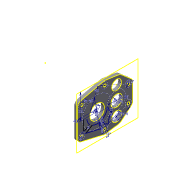
# Autodesk Inventor part: BackPlate
Saved by Autodesk Inventor 2013 SP1 (Build 170176100, 176)
## iProperties
Created: 2013-11-05
Part Number: BackPlate
Material: Generic
Document SubType Name: Modeling
Designer: robotics
Density: 1 g/cm^3
Author: robotics
Autodesk Inventor part; units mm, degrees
ref_plane "YZ Plane" through (0, 0, 0) normal (1, 0, 0) x (0, 1, 0)
ref_plane "XZ Plane" through (0, 0, 0) normal (0, 1, 0) x (-1, 0, 0)
ref_plane "XY Plane" through (0, 0, 0) normal (0, 0, 1) x (1, 0, 0)
sketch "Sketch1" plane through (0, 0, 0) normal (1, 0, 0) x (0, 1, 0)
  line L0 (181.2823, -83.3004) -> (61.2823, -83.3004)
  line L1 (61.2823, -83.3004) -> (61.2823, -183.3004)
  line L2 (61.2823, -183.3004) -> (181.2823, -183.3004)
  line L3 (181.2823, -183.3004) -> (181.2823, -83.3004)
  point P0 (0, 0)
  dimension "d0" = 100
  dimension "d2" = 120
  constraints: 8 end point, 2 parallel, 1 horizontal, 1 perpendicular, 1 other
  measures "d0" distance of L2.end L0.start
  measures "d2" distance of L0.start L0.end
extrude "Extrusion1" add sketch "Sketch1" along normal blind 6
sketch "Sketch2" plane through (6, 0, 0) normal (1, 0, 0) x (0, 0, -1)
  line L0 (83.3004, 181.2823) -> (83.3004, 61.2823) projected
  line L1 (83.3004, 61.2823) -> (183.3004, 61.2823) projected
  line L2 (183.3004, 61.2823) -> (183.3004, 181.2823) projected
  line L3 (183.3004, 181.2823) -> (83.3004, 181.2823) projected
  circle A0 centre (133.3004, 139.3823) radius 17.78 construction
  circle A1 centre (133.3004, 139.3823) radius 9.525 construction
  circle A2 centre (159.9704, 139.3823) radius 8.89 construction
  circle A3 centre (106.6304, 139.3823) radius 8.89 construction
  circle A4 centre (133.3004, 101.2823) radius 28.575 construction
  line L4 (159.9704, 139.3823) -> (149.536, 162.5401) construction
  line L5 (159.9704, 139.3823) -> (170.4047, 116.2245) construction
  line L6 (96.196, 116.2245) -> (106.6304, 139.3823) construction
  line L7 (106.6304, 139.3823) -> (117.0647, 162.5401) construction
  circle A5 centre (149.536, 162.5401) radius 6.35 construction
  circle A6 centre (170.4047, 116.2245) radius 6.35 construction
  circle A7 centre (96.196, 116.2245) radius 6.35 construction
  circle A8 centre (117.0647, 162.5401) radius 6.35 construction
  circle A9 centre (159.9704, 71.471) radius 6.35 construction
  circle A10 centre (106.6304, 71.471) radius 6.35 construction
  point P0 (0, 0)
  dimension "d5" = 35.56
  dimension "d7" = 19.05
  dimension "d8" = 57.15
  dimension "d9" = 17.78
  dimension "d10" = 25.4
  dimension "d11" = 12.7
  dimension "d12" = 40
  dimension "d13" = 40
  dimension "d14" = 50
  dimension "d22" = 40
  constraints: 11 centre point, 8 end point, 6 equal radius, 5 coincident, 4 horizontal alignment, 3 equal length, 3 tangent, 3 vertical alignment, 2 collinear
  measures "d5" diameter of A0
  measures "d7" diameter of A1
  measures "d8" diameter of A4
  measures "d9" diameter of A2
  measures "d10" distance of L4.start L4.end
  measures "d11" diameter of A8
  measures "d12" distance of A4.centre A7.centre
  measures "d13" distance from line of A4.centre L1
  measures "d14" distance from line of L0 A4.centre
  measures "d22" distance of A4.centre A10.centre
sketch "Sketch3" plane through (6, 0, 0) normal (1, 0, 0) x (0, 0, -1)
  circle A0 centre (133.3004, 101.2823) radius 14.2875
  circle A1 centre (133.3004, 139.3823) radius 11.1125
  circle A2 centre (106.6304, 139.3823) radius 9.5631
  circle A3 centre (159.9704, 139.3823) radius 9.5631
  circle A4 centre (170.4047, 116.2245) radius 2.5
  circle A5 centre (149.536, 162.5401) radius 2.5
  circle A6 centre (117.0647, 162.5401) radius 2.5
  circle A7 centre (96.196, 116.2245) radius 2.5
  circle A8 centre (106.6304, 71.471) radius 2.5
  circle A9 centre (159.9704, 71.471) radius 2.5
  point P0 (0, 0)
  dimension "d15" = 22.225
  dimension "d17" = 28.575
  dimension "d18" = 19.1262
  dimension "d19" = 5
  constraints: 10 centre point, 10 coincident, 6 equal radius
  measures "d15" diameter of A1
  measures "d17" diameter of A0
  measures "d18" diameter of A2
  measures "d19" diameter of A4
extrude "Extrusion2" cut sketch "Sketch3" against normal blind 6
sketch "Sketch4" plane through (6, 0, 0) normal (1, 0, 0) x (0, 0, -1)
  circle A0 centre (133.3004, 139.3823) radius 11.1125 projected
  circle A1 centre (170.4047, 116.2245) radius 2.5 projected
  circle A2 centre (149.536, 162.5401) radius 2.5 projected
  circle A3 centre (159.9704, 139.3823) radius 9.5631 projected
  circle A4 centre (133.3004, 101.2823) radius 14.2875 projected
  line L0 (83.3004, 181.2823) -> (83.3004, 61.2823) projected
  line L1 (83.3004, 61.2823) -> (183.3004, 61.2823) projected
  line L2 (183.3004, 61.2823) -> (183.3004, 181.2823) projected
  line L3 (183.3004, 181.2823) -> (83.3004, 181.2823) projected
  circle A5 centre (106.6304, 71.471) radius 2.5 projected
  circle A6 centre (159.9704, 71.471) radius 2.5 projected
  arc A7 (159.9704, 62.971) -> (168.2483, 69.541) centre (159.9704, 71.471) ccw
  arc A8 (178.6827, 114.2944) -> (178.8197, 117.4236) centre (170.4047, 116.2245) ccw
  arc A9 (175.3778, 141.5778) -> (171.8222, 149.4691) centre (159.9704, 139.3823) ccw
  arc A10 (156.0091, 168.0492) -> (149.536, 171.0401) centre (149.536, 162.5401) ccw
  line L4 (168.2483, 69.541) -> (178.6827, 114.2944)
  line L5 (178.8197, 117.4236) -> (175.3778, 141.5778)
  line L6 (171.8222, 149.4691) -> (156.0091, 168.0492)
  line L7 (149.536, 171.0401) -> (133.3004, 171.0401)
  line L8 (159.9704, 62.971) -> (133.3004, 62.971)
  line L9 (133.3004, 139.3823) -> (133.3004, 101.2823) construction
  arc A11 (98.3524, 69.541) -> (106.6304, 62.971) centre (106.6304, 71.471) ccw
  arc A12 (87.781, 117.4236) -> (87.918, 114.2944) centre (96.196, 116.2245) ccw
  arc A13 (94.7785, 149.4691) -> (91.2229, 141.5778) centre (106.6304, 139.3823) ccw
  arc A14 (117.0647, 171.0401) -> (110.5917, 168.0492) centre (117.0647, 162.5401) ccw
  line L10 (98.3524, 69.541) -> (87.918, 114.2944)
  line L11 (87.781, 117.4236) -> (91.2229, 141.5778)
  line L12 (94.7785, 149.4691) -> (110.5917, 168.0492)
  line L13 (117.0647, 171.0401) -> (133.3004, 171.0401)
  line L14 (106.6304, 62.971) -> (133.3004, 62.971)
  point P0 (0, 0)
  dimension "d23" = 6
  dimension "d24" = 6
  constraints: 22 end point, 16 point on circle, 12 symmetric about line, 8 centre point, 8 tangent, 4 coincident, 2 equal radius, 2 parallel, 2 vertical alignment, 1 perpendicular, 4 other
  measures "d23" radial gap between concentric circles of A7 A6
  measures "d24" radial gap between concentric circles of A3 A9
extrude "Extrusion3" cut sketch "Sketch4" against normal blind 6 contours L3 L2 L1 L0
sketch "Sketch7" plane through (6, 0, 0) normal (1, 0, 0) x (0, 0, -1)
  line L0 (168.2483, 69.541) -> (178.6827, 114.2944) projected
  arc A0 (178.6827, 114.2944) -> (178.8197, 117.4236) centre (170.4047, 116.2245) ccw projected
  line L1 (178.8197, 117.4236) -> (175.3778, 141.5778) projected
  arc A1 (175.3778, 141.5778) -> (171.8222, 149.4691) centre (159.9704, 139.3823) ccw projected
  line L2 (171.8222, 149.4691) -> (156.0091, 168.0492) projected
  arc A2 (156.0091, 168.0492) -> (149.536, 171.0401) centre (149.536, 162.5401) ccw projected
  line L3 (149.536, 171.0401) -> (117.0647, 171.0401) projected
  arc A3 (117.0647, 171.0401) -> (110.5917, 168.0492) centre (117.0647, 162.5401) ccw projected
  line L4 (110.5917, 168.0492) -> (94.7785, 149.4691) projected
  arc A4 (94.7785, 149.4691) -> (91.2229, 141.5778) centre (106.6304, 139.3823) ccw projected
  line L5 (91.2229, 141.5778) -> (87.781, 117.4236) projected
  arc A5 (87.781, 117.4236) -> (87.918, 114.2944) centre (96.196, 116.2245) ccw projected
  line L6 (87.918, 114.2944) -> (98.3524, 69.541) projected
  arc A6 (98.3524, 69.541) -> (106.6304, 62.971) centre (106.6304, 71.471) ccw projected
  line L7 (106.6304, 62.971) -> (159.9704, 62.971) projected
  arc A7 (159.9704, 62.971) -> (168.2483, 69.541) centre (159.9704, 71.471) ccw projected
  circle A8 centre (133.3004, 139.3823) radius 11.1125 projected
  circle A9 centre (106.6304, 139.3823) radius 9.5631 projected
  circle A10 centre (106.6304, 71.471) radius 2.5 projected
  circle A11 centre (117.0647, 162.5401) radius 2.5 projected
  circle A12 centre (170.4047, 116.2245) radius 2.5 projected
  circle A13 centre (149.536, 162.5401) radius 2.5 projected
  circle A14 centre (96.196, 116.2245) radius 2.5 projected
  circle A15 centre (159.9704, 71.471) radius 2.5 projected
  circle A16 centre (159.9704, 139.3823) radius 9.5631 projected
  circle A17 centre (133.3004, 101.2823) radius 14.2875 projected
  arc A18 (153.2129, 76.6273) -> (151.9321, 74.2344) centre (159.9704, 71.471) ccw
  arc A19 (158.8545, 79.8975) -> (158.3019, 79.8057) centre (159.9704, 71.471) ccw
  arc A20 (164.1481, 110.4708) -> (165.6772, 109.1604) centre (170.4047, 116.2245) ccw
  arc A21 (164.4024, 122.243) -> (161.9068, 116.0364) centre (170.4047, 116.2245) ccw
  arc A22 (147.5845, 129.9589) -> (163.5086, 124.2267) centre (159.9704, 139.3823) ccw
  arc A23 (136.3004, 122.5348) -> (147.5845, 129.9589) centre (133.3004, 139.3823) ccw
  arc A24 (150.7916, 111.5603) -> (136.3004, 121.3467) centre (133.3004, 101.2823) ccw
  arc A25 (151.0381, 91.4358) -> (153.033, 105.9946) centre (133.3004, 101.2823) ccw
  arc A26 (135.4738, 81.1115) -> (147.1014, 86.4124) centre (133.3004, 101.2823) ccw
  line L8 (153.2129, 76.6273) -> (147.1014, 86.4124)
  line L9 (151.9321, 74.2344) -> (132.9586, 74.2344)
  line L10 (165.6772, 109.1604) -> (158.8545, 79.8975)
  line L11 (158.3019, 79.8057) -> (151.0381, 91.4358)
  line L12 (153.033, 105.9946) -> (164.1481, 110.4708)
  line L13 (161.9068, 116.0364) -> (150.7916, 111.5603)
  line L14 (136.3004, 121.3467) -> (136.3004, 122.5348)
  line L15 (163.5086, 124.2267) -> (164.4024, 122.243)
  point P0 (0, 0)
  dimension "d27" = 6
  dimension "d28" = 6
  dimension "d29" = 6
  dimension "d30" = 6
  dimension "d31" = 6
  dimension "d32" = 6
  dimension "d33" = 3
  dimension "d34" = 3
  dimension "d35" = 3
  dimension "d36" = 3
  dimension "d37" = 3
  dimension "d38" = 3
  dimension "d39" = 3
  constraints: 19 point on circle, 16 end point, 9 centre point, 9 coincident, 5 equal radius, 4 parallel, 1 vertical
  measures "d27" radial gap between concentric circles of A22 A16
  measures "d28" radial gap between concentric circles of A8 A23
  measures "d29" radial gap between concentric circles of A17 A24
  measures "d30" radial gap between concentric circles of A12 A20
  measures "d31" distance between parallel lines of L12 L13
  measures "d32" distance between parallel lines of L8 L11
  measures "d33" distance from line of A17.centre L14
  measures "d34" distance from line of A7.centre L10
  measures "d35" distance from line of A0.centre L13
  measures "d36" distance from line of A17.centre L12
  measures "d37" distance from line of A0.centre L15
  measures "d38" distance from line of A1.centre L15
  measures "d39" distance from line of A7.centre L11
equation "\"d22\" = d12"
body "Solid1"
